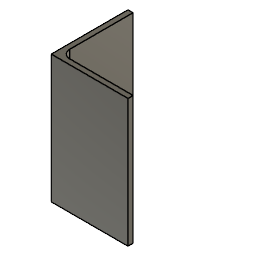
L-60×60×4 (Autodesk Fusion 360 design; units mm, degrees)
Autodesk Fusion 360 part; units mm, degrees
note: some values were not read from the file. Set by a fixed rule: which sketch regions a step uses.
sketch "スケッチ1" plane through (0, 0, 0) normal (0, 0, 1) x (1, 0, 0)
  line L0 (0, 60) -> (0, 0)
  line L1 (4, 10.5) -> (4, 60)
  line L2 (60, 4) -> (10.5, 4)
  line L3 (0, 0) -> (60, 0)
  arc A0 (4, 10.5) -> (10.5, 4) centre (10.5, 10.5) ccw
  line L4 (60, 0) -> (60, 4)
  line L5 (4, 60) -> (0, 60)
extrude "押し出し1" add sketch "スケッチ1" along normal blind 100
